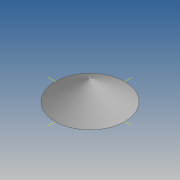
# Autodesk Inventor part: P023_Chapeau
Saved by Autodesk Inventor 2021.3 (Build 253353000, 353)
## iProperties
Created: 2021-11-18
Part Number: P023_Chapeau
Material: Générique
Document SubType Name: Modeling
Designer: gabri
Density: 1 g/cm^3
Appearance: Par défaut
Author: gabri
Autodesk Inventor part; units mm, degrees
ref_plane "YZ Plane" through (0, 0, 0) normal (1, 0, 0) x (0, 1, 0)
ref_plane "XZ Plane" through (0, 0, 0) normal (0, 1, 0) x (-1, 0, 0)
ref_plane "XY Plane" through (0, 0, 0) normal (0, 0, 1) x (1, 0, 0)
sketch "Sketch2" plane through (0, 0, 0) normal (0, 1, 0) x (-1, 0, 0)
  line L0 (0, 103.923) -> (-180, 0)
  line L1 (36, 0) -> (-216, 0) construction
  line L2 (0, -74.1996) -> (0, 263.8391) construction
  line L3 (0, 103.923) -> (0, 101.6136)
  line L4 (0, 101.6136) -> (-176, 0)
  line L5 (-180, 0) -> (-176, 0)
  line L6 (0, 215.5479) -> (0, -25.9084)
  point P0 (0, 0)
  dimension "d0" = 180
  dimension "d3" = 30
  dimension "d4" = 2
  constraints: 10 end point, 6 point on line, 1 collinear, 1 parallel
  measures "d0" distance of L0.end point (0, 0)
  measures "d3" angle of L1 L0
  measures "d4" distance between parallel lines of L0 L4
revolve "Revolution1" add sketch "Sketch2" angle 360 about axis through (0, 0, 215.5479) along (0, 0, -1)
body "Solid1"
